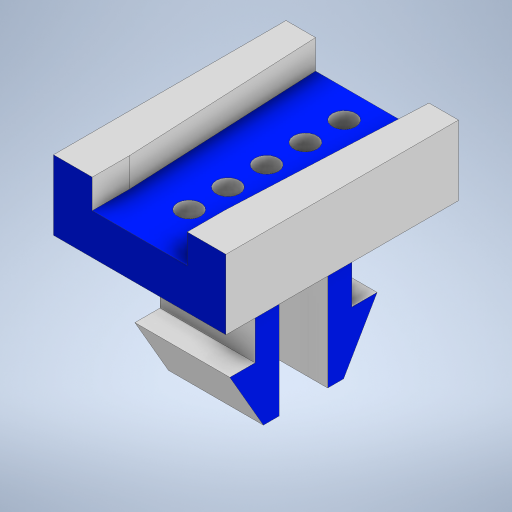
# Autodesk Inventor part: PlugConnectionBigServo
Saved by Autodesk Inventor 2023 (Build 270158000, 158)
## iProperties
Created: 2023-07-17
Part Number: PlugConnectionBigServo
Material: Generic
Document SubType Name: Modeling
Designer: Admin
Density: 1 g/cm^3
Appearance: Default
Author: Admin
Autodesk Inventor part; units mm, degrees
ref_plane "YZ Plane" through (0, 0, 0) normal (1, 0, 0) x (0, 1, 0)
ref_plane "XZ Plane" through (0, 0, 0) normal (0, 1, 0) x (-1, 0, 0)
ref_plane "XY Plane" through (0, 0, 0) normal (0, 0, 1) x (1, 0, 0)
sketch "Sketch1" plane through (0, 0, 0) normal (0, 1, 0) x (-1, 0, 0)
  circle A0 centre (0, 0) radius 1.75
  circle A1 centre (0, 0) radius 2.45
  line L0 (0.95, 1.4697) -> (0.95, -1.4697)
  line L1 (1.5, 13) -> (-1.5, 13) construction
  line L2 (-1.5, 13) -> (-1.5, 5) construction
  line L3 (-1.5, 5) -> (1.5, 5) construction
  line L4 (1.5, 5) -> (1.5, 13) construction
  line L5 (0, 5) -> (0, 0) construction
  line L6 (2.45, 0) -> (2.45, 15)
  line L7 (2.45, 15) -> (-2.45, 15)
  line L8 (-2.45, 15) -> (-2.45, 0)
  line L9 (2.45, 0) -> (2.45, -2)
  line L10 (0.45, -4) -> (-0.45, -4)
  line L11 (-2.45, -2) -> (-2.45, 0)
  arc A2 (0.45, -4) -> (2.45, -2) centre (0.45, -2) ccw
  arc A3 (-2.45, -2) -> (-0.45, -4) centre (-0.45, -2) ccw
  line L12 (2.45, 3) -> (-2.45, 3)
  dimension "d0" = 3.5
  dimension "d1" = 4.9
  dimension "d3" = 3
  dimension "d4" = 8
  dimension "d5" = 5
  dimension "d6" = 2
  dimension "d15" = 2.7
  dimension "d24" = 4
  dimension "d25" = 2
  dimension "d28" = 2
  constraints: 26 end point, 8 point on circle, 7 tangent, 6 vertical, 4 centre point, 4 perpendicular, 2 coincident, 2 parallel, 2 point on line, 1 equal radius, 1 horizontal, 1 midpoint
  measures "d0" diameter of A0
  measures "d1" diameter of A1
  measures "d3" distance between parallel lines of L2 L4
  measures "d4" distance between parallel lines of L1 L3
  measures "d5" distance from line of point (0, 0) L3
  measures "d6" distance between parallel lines of L7 L1
  measures "d24" distance from line of L10 point (0, 0)
  measures "d25" radius of A2
  measures "d28" distance between parallel lines of L12 L3
extrude "Extrusion1" add sketch "Sketch1" along normal blind 2.1 contours L12 L8 L7 L6
sketch "Sketch2" plane through (0, 0, 0) normal (0, -1, 0) x (1, 0, 0)
  line L0 (2.45, 12.8) -> (-2.45, 12.8)
  line L1 (-2.45, 12.8) -> (-2.45, 5.2)
  line L2 (-2.45, 5.2) -> (2.45, 5.2)
  line L3 (2.45, 5.2) -> (2.45, 12.8)
  line L4 (0, 0) -> (0, 5.2) construction
  line L5 (2.45, 9) -> (-2.45, 9) construction
  line L6 (-2.45, 15) -> (2.45, 15) projected
  line L7 (2.45, 15) -> (2.45, 3) projected
  dimension "d10" = 7.6
  constraints: 12 end point, 4 midpoint, 3 parallel, 1 horizontal, 1 perpendicular, 1 point on line, 1 vertical
  measures "d10" distance between parallel lines of L0 L2
extrude "Extrusion2" add sketch "Sketch2" along normal blind 7
sketch "Sketch3" plane through (2.45, 0, -3) normal (1, 0, 0) x (0, 0, -1)
  line L0 (-15.8, 0) -> (-15.8, -7) projected
  line L1 (-15.8, -4) -> (-14.0679, -7)
  line L2 (-13.25, -7) -> (-13.25, 0)
  line L3 (-13.25, 0) -> (-10.75, 0)
  line L4 (-10.75, 0) -> (-10.75, -7)
  line L5 (-10.75, -7) -> (-9.9321, -7)
  line L6 (-9.9321, -7) -> (-8.2, -4)
  line L7 (-8.2, -4) -> (-9.5, -4)
  line L8 (-9.5, -4) -> (-9.5, 0)
  line L9 (-8.2, 0) -> (-8.2, -7) projected
  line L10 (-9.5, 0) -> (-8.2, 0)
  line L11 (-13.25, -7) -> (-14.0679, -7)
  line L12 (-15.8, -4) -> (-14.5, -4)
  line L13 (-14.5, -4) -> (-14.5, 0)
  line L14 (-14.5, 0) -> (-15.8, 0)
  line L15 (-13.25, -7) -> (-12, -6.9306) construction
  line L16 (-10.75, -7) -> (-13.25, -7)
  line L17 (-8.2, -7) -> (-15.8, -7) projected
  line L18 (-15.8, 0) -> (-15.8, -7) projected
  line L19 (-15.8, -4) -> (-15.8, -7)
  line L20 (-15.8, -7) -> (-14.0679, -7)
  line L21 (-3, 0) -> (-8.2, 0) projected
  line L22 (-8.2, 0) -> (-8.2, -4)
  line L23 (-12, -6.9306) -> (-12, 0) construction
  line L24 (-9.5, -4) -> (-10.75, -4) construction
  line L25 (-14.5, -4) -> (-13.25, -4) construction
  line L26 (-6, 0) -> (-18, 0) projected
  line L27 (-17.9, 0) -> (-18, 0)
  line L28 (-18, 0) -> (-6, 0) projected
  line L29 (-6.1, 0) -> (-6, 0)
  point P0 (-9.9321, -7)
  point P1 (-18, 2.1)
  point P2 (-6, 2.1)
  point P3 (-18.8, 0)
  point P4 (-14.75, -6.5676)
  point P5 (-12.25, -5.8187)
  point P6 (-10.75, -7)
  dimension "d18" = 4
  dimension "d19" = 1.25
  dimension "d20" = 1.25
  dimension "d22" = 60
  constraints: 46 end point, 7 perpendicular, 6 collinear, 6 point on line, 5 vertical, 3 horizontal, 1 midpoint, 4 other
  measures "d18" distance between parallel lines of L10 L7
  measures "d19" distance between parallel lines of L13 L2
  measures "d20" distance between parallel lines of L23 L4
  measures "d22" angle of L7 L6
extrude "Extrusion5" cut sketch "Sketch3" against normal up to surface (4.9 mm away) contours L14 L13 L12 L0 | L1 L17 L0 | L3 L4 L16 L2 | L10 L9 L7 L8 | L6 L9 L17
sketch "Sketch5" plane through (0, 2.1, 0) normal (0, 1, 0) x (1, 0, 0)
  circle A0 centre (0, 0) radius 1.05
  circle A1 centre (0, 0) radius 3.45
  line L0 (2.3973, -14.1638) -> (2.9878, -1.725)
  line L1 (2.9878, -1.725) -> (2.3973, -14.1638)
  arc A2 (-2.3973, -14.1638) -> (2.3973, -14.1638) centre (0, -14.05) ccw
  line L2 (-2.3973, -14.1638) -> (-2.9878, -1.725)
  arc A3 (-2.3973, -14.1638) -> (2.3973, -14.1638) centre (0, -14.05) ccw
  circle A4 centre (0, -4.45) radius 0.25
  circle A5 centre (0, -4.45) radius 0.6 construction
  circle A6 centre (0, -6.45) radius 0.6 construction
  circle A7 centre (0, -6.45) radius 0.25
  circle A8 centre (0, -8.45) radius 0.25
  circle A9 centre (0, -8.45) radius 0.6 construction
  circle A10 centre (0, -10.45) radius 0.25
  circle A11 centre (0, -10.45) radius 0.6 construction
  circle A12 centre (0, -12.45) radius 0.25
  circle A13 centre (0, -12.45) radius 0.6 construction
  circle A14 centre (0, -14.45) radius 0.25
  circle A15 centre (0, -14.45) radius 0.6 construction
  line L3 (0, -11.65) -> (0, 0) construction
  line L4 (0, -4.45) -> (0, -6.45)
  line L5 (0, -6.45) -> (0, -8.45)
  line L6 (0, -8.45) -> (0, -10.45)
  line L7 (0, -10.45) -> (0, -12.45)
  line L8 (0, -12.45) -> (0, -14.45)
  line L9 (0, 0) -> (-2.9878, -1.725) construction
  line L10 (0, 0) -> (2.9878, -1.725) construction
  line L11 (-2.9878, -1.725) -> (0, -1.725) construction
  line L12 (2.9878, -1.725) -> (0, -1.725) construction
  line L13 (-4.45, -3) -> (4.45, -3)
  line L14 (4.45, -3) -> (4.45, -15)
  line L15 (4.45, -15) -> (-4.45, -15)
  line L16 (-4.45, -15) -> (-4.45, -3)
  line L17 (-2.45, -3) -> (-2.45, -15) projected
  line L18 (2.45, -15) -> (2.45, -3) projected
  line L19 (-2.45, -15) -> (2.45, -15) projected
  line L20 (2.45, -3) -> (-2.45, -3) projected
  point P0 (2.45, -13.0537)
  point P1 (2.204, -15)
  point P2 (-2.204, -15)
  point P3 (-2.45, -13.0537)
  point P4 (-2.9273, -3)
  point P5 (2.9273, -3)
  dimension "d34" = 2.1
  dimension "d35" = 6.9
  dimension "d36" = 2
  dimension "d37" = 0.5
  dimension "d38" = 2.4
  dimension "d39" = 0.4
  dimension "d41" = 60
  dimension "d42" = 4.45
  dimension "d43" = 2
  dimension "d44" = 2
  dimension "d49" = 1.2
  constraints: 32 end point, 16 centre point, 10 collinear, 10 equal radius, 8 coincident, 8 point on circle, 3 vertical, 2 horizontal, 2 parallel, 1 concentric, 1 perpendicular, 1 tangent, 12 other
  measures "d34" diameter of A0
  measures "d35" diameter of A1
  measures "d36" distance of A7.centre A5.centre
  measures "d37" diameter of A4
  measures "d38" radius of A3
  measures "d39" distance of A15.centre A2.centre
  measures "d41" angle to the sketch y axis of L9
  measures "d42" distance of A0.centre L4.start
  measures "d43" distance between parallel lines of L16 L17
  measures "d44" distance between parallel lines of L18 L14
  measures "d49" diameter of A5
extrude "Extrusion6" add sketch "Sketch5" along normal blind 1.5 and the other way blind 2.1 contours L2 L17 L15 L16 L13 | L13 L14 L15 L18 L0
sketch "Sketch7" plane through (0, 2.1, 0) normal (0, 1, 0) x (1, 0, 0)
  line L0 (-2.9273, -3) -> (-4.45, -3) projected
  line L1 (4.45, -15) -> (4.45, -3) projected
  line L2 (-4.45, -3) -> (4.45, -3)
  line L3 (4.45, -3) -> (4.45, -15)
  line L4 (4.45, -15) -> (-4.45, -15)
  line L5 (-4.45, -15) -> (-4.45, -3)
  point P0 (0, 0)
  point P1 (4.45, -3)
  constraints: 8 end point, 2 parallel, 1 horizontal, 1 perpendicular
extrude "Extrusion8" add sketch "Sketch7" against normal blind 2.1
sketch "Sketch6" plane through (0, 2.1, 0) normal (0, 1, 0) x (1, 0, 0)
  circle A0 centre (0, 0) radius 1.05
  circle A1 centre (0, 0) radius 3.45
  circle A2 centre (0, -14.45) radius 0.6
  circle A3 centre (0, -14.45) radius 0.6 construction
  arc A4 (-1.997, -14.1591) -> (1.997, -14.1591) centre (0, -14.05) ccw
  arc A5 (-1.997, -14.1591) -> (1.997, -14.1591) centre (0, -14.05) ccw
  circle A6 centre (0, -4.45) radius 0.6
  circle A7 centre (0, -4.45) radius 0.6 construction
  circle A8 centre (0, -6.45) radius 0.6
  circle A9 centre (0, -8.45) radius 0.6
  circle A10 centre (0, -8.45) radius 0.6 construction
  line L0 (1.997, -14.1591) -> (2.65, -2.2091)
  line L1 (2.65, -2.2091) -> (1.997, -14.1591)
  line L2 (-1.997, -14.1591) -> (-2.65, -2.2091)
  circle A11 centre (0, -10.45) radius 0.6
  circle A12 centre (0, -10.45) radius 0.6 construction
  circle A13 centre (0, -12.45) radius 0.6
  circle A14 centre (0, -12.45) radius 0.6 construction
  circle A15 centre (0, -6.45) radius 0.6 construction
  line L3 (0, -12.05) -> (0, 0) construction
  line L4 (0, -4.45) -> (0, -6.45)
  line L5 (0, -6.45) -> (0, -8.45)
  line L6 (0, -8.45) -> (0, -10.45)
  line L7 (0, -10.45) -> (0, -12.45)
  line L8 (0, -12.45) -> (0, -14.45)
  line L9 (0, 0) -> (-2.65, -2.2091) construction
  line L10 (0, 0) -> (2.65, -2.2091) construction
  line L11 (-2.65, -2.2091) -> (0, -2.2091) construction
  line L12 (2.65, -2.2091) -> (0, -2.2091) construction
  line L13 (-4.45, -3) -> (4.45, -3)
  line L14 (4.45, -3) -> (4.45, -15)
  line L15 (4.45, -15) -> (-4.45, -15)
  line L16 (-4.45, -15) -> (-4.45, -3)
  line L17 (-2.45, -3) -> (-2.45, -15)
  line L18 (2.45, -15) -> (2.45, -3)
  line L19 (-2.45, -15) -> (2.45, -15)
  line L20 (2.45, -3) -> (-2.45, -3)
  point P0 (-0.2398, -15)
  point P1 (0.2398, -15)
  dimension "d50" = 2.1
  dimension "d51" = 6.9
  dimension "d52" = 2
  dimension "d53" = 1.2
  dimension "d54" = 2
  dimension "d55" = 0.4
  dimension "d56" = 50.185
  dimension "d57" = 4.45
  dimension "d58" = 2
  dimension "d59" = 2
  dimension "d60" = 1.2
  constraints: 40 end point, 16 centre point, 10 collinear, 10 equal radius, 9 coincident, 8 point on circle, 3 vertical, 2 horizontal, 2 parallel, 1 concentric, 1 perpendicular, 1 tangent, 12 other
  measures "d50" diameter of A0
  measures "d51" diameter of A1
  measures "d52" distance of A8.centre A7.centre
  measures "d53" diameter of A6
  measures "d54" radius of A4
  measures "d55" distance of A3.centre A5.centre
  measures "d56" angle to the sketch y axis of L9
  measures "d57" distance of A0.centre L4.start
  measures "d58" distance between parallel lines of L16 L17
  measures "d59" distance between parallel lines of L18 L14
  measures "d60" diameter of A7
extrude "Extrusion7" cut sketch "Sketch6" against normal blind 1.5 contours A6 | A8 L4 L5 | L5 L4 A8 | A9 L5 L6 | L6 L5 A9 | A11 L6 L7 | L7 L6 A11 | A13 L7 L8 | L8 L7 A13
body "Solid1"
